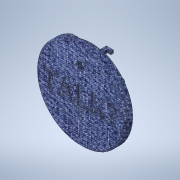
# Autodesk Inventor part: ButtonCap
Saved by Autodesk Inventor 2020.1 (Build 241239000, 239)
## iProperties
Created: 2019-10-05
Part Number: ButtonCap
Material: Plastic, Opaque Black
Document SubType Name: Modeling
Designer: Josiah
Density: 0.952 g/cm^3
Appearance: Denim - Blue
Author: Josiah
Autodesk Inventor part; units mm, degrees
ref_plane "YZ Plane" through (0, 0, 0) normal (1, 0, 0) x (0, 1, 0)
ref_plane "XZ Plane" through (0, 0, 0) normal (0, 1, 0) x (-1, 0, 0)
ref_plane "XY Plane" through (0, 0, 0) normal (0, 0, 1) x (1, 0, 0)
sketch "Sketch2" plane through (0, 0, 0) normal (0, 0, 1) x (1, 0, 0)
  arc A0 (-10.102, 26.1034) -> (10.102, 26.1034) centre (0, 0) ccw construction
  circle A1 centre (0, 0) radius 24.99 construction
  circle A2 centre (0, 0) radius 27.99
  constraints: 2 coincident, 1 centre point, 1 concentric, 3 other
extrude "BUTTON TOP" add sketch "Sketch2" along normal blind 3
chamfer "BUTTON TOP CHAMFER" distance 1 angle 45 1 edges at (-27.99, 0, 3)
sketch "Sketch3" plane through (0, 0, 0) normal (0, 0, -1) x (-1, 0, 0)
  circle A0 centre (0, 0) radius 24.99 projected
  line L0 (-10.102, 26.1034) -> (10.102, 26.1034) projected
  arc A1 (-10.102, 26.1034) -> (10.102, 26.1034) centre (0, 0) ccw projected
  point P0 (0, 0)
extrude "WALLS" add sketch "Sketch3" along normal blind 1.9
sketch "Sketch4" plane through (0, 0, 0) normal (0, 0, -1) x (-1, 0, 0)
  circle A0 centre (0, 0) radius 24.99 projected
  circle A1 centre (0, 0) radius 21.99
  point P0 (0, 0)
  dimension "d9" = 3
  constraints: 1 centre point
  measures "d9" radial gap between concentric circles of A0 A1
extrude "INNTER SHEATH" add sketch "Sketch4" along normal blind 4
sketch "Sketch5" plane through (0, 0, 0) normal (0, 0, -1) x (-1, 0, 0)
  circle A0 centre (0, 0) radius 3.5 construction
  circle A1 centre (0, 0) radius 4
  point P0 (0, 0)
  dimension "d12" = 0.5
  constraints: 1 centre point
  measures "d12" radial gap between concentric circles of A0 A1
extrude "BUTTON INDENT" cut sketch "Sketch5" against normal blind 1
sketch "Sketch6" plane through (0, 0, 0) normal (0, 0, -1) x (-1, 0, 0)
  circle A0 centre (-15, 10) radius 2.5 construction
  circle A1 centre (15, 10) radius 2.5 construction
  circle A2 centre (15, -10) radius 2.5 construction
  circle A3 centre (-15, -10) radius 2.5 construction
  circle A4 centre (-15, 10) radius 2.4
  circle A5 centre (15, 10) radius 2.4
  circle A6 centre (15, -10) radius 2.4
  circle A7 centre (-15, -10) radius 2.4
  point P0 (0, 0)
  dimension "d15" = 0.1
  dimension "d16" = 0.1
  dimension "d17" = 0.1
  dimension "d18" = 0.1
  constraints: 4 centre point
  measures "d15" radial gap between concentric circles of A1 A5
  measures "d16" radial gap between concentric circles of A2 A6
  measures "d17" radial gap between concentric circles of A3 A7
  measures "d18" radial gap between concentric circles of A0 A4
extrude "BUTTON-PINS" add sketch "Sketch6" along normal blind 8
fillet "PIN-FILLET" radius 0.5 4 edges at (17.4, 10, -8) (-12.6, 10, -8) (17.4, -10, -8) (-12.6, -10, -8)
sketch "Sketch7" plane through (0, 0, 0) normal (0, 0, -1) x (-1, 0, 0)
  line L0 (-9, 21.1034) -> (-8.5703, 21.1034) construction
  line L1 (-8.5703, 21.1034) -> (-6.6338, 21.1034) construction
  line L2 (-6.6338, 21.1034) -> (-5.6655, 21.1034) construction
  line L3 (-5.6655, 21.1034) -> (-4.602, 21.1034) construction
  circle A0 centre (0, 0) radius 24.99 construction
  line L4 (-9, 23.3131) -> (-9, 21.1034) construction
  line L5 (-8.702, 21.2034) -> (-4.302, 21.2034)
  line L6 (-4.302, 21.2034) -> (-4.302, 23.2034)
  line L7 (-4.302, 23.2034) -> (-8.702, 23.2034)
  line L8 (-8.702, 23.2034) -> (-8.702, 21.2034)
  point P0 (0, 0)
  dimension "d22" = 2
  dimension "d23" = 4.4
  dimension "d24" = 0.1
  dimension "d25" = 0.3
  constraints: 8 end point, 2 parallel, 1 horizontal, 1 perpendicular, 1 other
  measures "d22" distance of L5.end L6.end
  measures "d23" distance of L6.end L7.end
  measures "d24" distance between parallel lines of L5 L3
  measures "d25" distance from line of L6 L3.end
extrude "LOCK BLOCK" add sketch "Sketch7" along normal blind 9
sketch "Sketch8" plane through (4.302, 23.2034, -4) normal (0, 1, 0) x (1, 0, 0)
  line L0 (4.4, 0) -> (0, 0) projected
  line L1 (4.4, 0) -> (4.4, 5) projected
  line L2 (0, 5) -> (4.4, 5) projected
  line L3 (0, 0) -> (0, 5) projected
  line L4 (4.4, 3.5) -> (2.2, 3.5)
  line L5 (2.2, 3.5) -> (2.2, 0)
  line L6 (2.2, 0) -> (4.4, 0)
  line L7 (4.4, 0) -> (4.4, 3.5)
  circle A0 centre (3.3, 2.4) radius 1 construction
  circle A1 centre (3.3, 2.4) radius 0.9
  point P0 (-4.302, -4)
  dimension "d28" = 0.1
  dimension "d29" = 0.2
  dimension "d32" = 0.2
  dimension "d33" = 1.5
  dimension "d44" = 0
  constraints: 8 end point, 2 parallel, 1 centre point, 1 horizontal, 1 perpendicular
  measures "d28" radial gap between concentric circles of A0 A1
  measures "d29" distance edge to line of A1 L5
  measures "d32" distance edge to line of A1 L4
  measures "d33" distance edge to line of A1 L6
  measures "d44" distance between parallel lines of L1 L7
extrude "LOCK HOLE" cut sketch "Sketch8" against normal up to next contours L0 L5 L4 L1 | A1
fillet "LOCK HOLE FILLET" radius 0.2 2 edges at (6.502, 22.2034, -7.5) (6.502, 22.2034, -4)
sketch "Sketch9" plane through (0, 0, 3) normal (0, 0, 1) x (1, 0, 0)
  circle A0 centre (0, 16) radius 2.5
  point P0 (0, 0)
  point P1 (0, 0)
  dimension "d37" = 5
  dimension "d38" = 0
  dimension "d39" = 16
  constraints: 1 centre point, 1 coincident, 2 other
  measures "d37" diameter of A0
  measures "d38" horizontal distance of point (0, 0) A0.centre
  measures "d39" distance of A0.centre point (0, 0)
extrude "LED HOLE" cut sketch "Sketch9" against normal up to next
sketch "Sketch10" plane through (0, 0, 3) normal (0, 0, 1) x (1, 0, 0)
  circle A0 centre (0, 16) radius 2.5 projected
  circle A1 centre (0, 0) radius 26.99 projected
  line L0 (-23.4481, 5.4662) -> (19.1517, 5.4662) construction
  line L1 (19.1517, 5.4662) -> (19.1517, -6.0554) construction
  line L2 (19.1517, -6.0554) -> (-23.4481, -6.0554) construction
  line L3 (-23.4481, -6.0554) -> (-23.4481, 5.4662) construction
  line L4 (-20.1058, -6.0627) -> (-20.1058, 3.0854)
  line L5 (-20.1058, 3.0854) -> (-23.4481, 3.0854)
  line L6 (-23.4481, 3.0854) -> (-23.4481, 5.2373)
  line L7 (-23.4481, 5.2373) -> (-13.9246, 5.2373)
  line L8 (-13.9246, 5.2373) -> (-13.9246, 3.0854)
  line L9 (-13.9246, 3.0854) -> (-17.267, 3.0854)
  line L10 (-17.267, 3.0854) -> (-17.267, -6.0627)
  line L11 (-17.267, -6.0627) -> (-20.1058, -6.0627)
  line L12 (-13.9796, -6.0627) -> (-10.161, 5.2373)
  line L13 (-10.161, 5.2373) -> (-7.0659, 5.2373)
  line L14 (-7.0659, 5.2373) -> (-3.2473, -6.0627)
  line L15 (-3.2473, -6.0627) -> (-6.1685, -6.0627)
  line L16 (-6.1685, -6.0627) -> (-6.8736, -3.7551)
  line L17 (-6.8736, -3.7551) -> (-10.4266, -3.7551)
  line L18 (-10.4266, -3.7551) -> (-11.1408, -6.0627)
  line L19 (-11.1408, -6.0627) -> (-13.9796, -6.0627)
  line L20 (-7.4963, -1.7039) -> (-8.6501, 2.0323)
  line L21 (-8.6501, 2.0323) -> (-9.813, -1.7039)
  line L22 (-9.813, -1.7039) -> (-7.4963, -1.7039)
  line L23 (5.4154, -6.0627) -> (-2.121, -6.0627)
  line L24 (-2.121, -6.0627) -> (-2.121, 5.2373)
  line L25 (-2.121, 5.2373) -> (0.7177, 5.2373)
  line L26 (0.7177, 5.2373) -> (0.7177, -3.9107)
  line L27 (0.7177, -3.9107) -> (5.4154, -3.9107)
  line L28 (5.4154, -3.9107) -> (5.4154, -6.0627)
  line L29 (16.6696, -6.0627) -> (13.2357, -6.0627)
  line L30 (13.2357, -6.0627) -> (10.168, -1.4749)
  line L31 (10.168, -1.4749) -> (9.6094, -2.2441)
  line L32 (9.6094, -2.2441) -> (9.6094, -6.0627)
  line L33 (9.6094, -6.0627) -> (6.7707, -6.0627)
  line L34 (6.7707, -6.0627) -> (6.7707, 5.2373)
  line L35 (6.7707, 5.2373) -> (9.6094, 5.2373)
  line L36 (9.6094, 5.2373) -> (9.6094, 0.1917)
  line L37 (9.6094, 0.1917) -> (13.2357, 5.2373)
  line L38 (13.2357, 5.2373) -> (16.5048, 5.2373)
  line L39 (16.5048, 5.2373) -> (12.4756, -0.0098)
  line L40 (12.4756, -0.0098) -> (16.6696, -6.0627)
  spline S0 degree 2 poles (24.6455, 2.481) (24.6455, 1.7301) (24.1968, 0.5397) (23.7848, 0.1001) knots 0 0 0 1 2 2 2
  spline S1 degree 2 poles (23.7848, 0.1001) (23.391, -0.3303) (22.2555, -1.0079) (21.5596, -1.2918) knots 0 0 0 1 2 2 2
  line L41 (21.5596, -1.2918) -> (21.5596, -3.0225)
  line L42 (21.5596, -3.0225) -> (18.9681, -3.0225)
  line L43 (18.9681, -3.0225) -> (18.9681, -0.4768)
  spline S2 degree 2 poles (18.9681, -0.4768) (19.3893, -0.3669) (20.4332, 0.0269) (20.827, 0.3107) knots 0 0 0 1 2 2 2
  spline S3 degree 2 poles (20.827, 0.3107) (21.2391, 0.6129) (21.7702, 1.4004) (21.7702, 1.9407) knots 0 0 0 1 2 2 2
  spline S4 degree 2 poles (21.7702, 1.9407) (21.7702, 2.6916) (20.8178, 3.3692) (19.9662, 3.3692) knots 0 0 0 1 2 2 2
  spline S5 degree 2 poles (19.9662, 3.3692) (19.3252, 3.3692) (17.8967, 2.8106) (17.4846, 2.5268) knots 0 0 0 1 2 2 2
  line L44 (17.4846, 2.5268) -> (17.2648, 2.5268)
  line L45 (17.2648, 2.5268) -> (17.2648, 4.8161)
  spline S6 degree 2 poles (17.2648, 4.8161) (17.7502, 5.0267) (19.6182, 5.4662) (20.6896, 5.4662) knots 0 0 0 1 2 2 2
  spline S7 degree 2 poles (20.6896, 5.4662) (21.642, 5.4662) (23.1071, 5.0175) (23.6199, 4.6146) knots 0 0 0 1 2 2 2
  spline S8 degree 2 poles (23.6199, 4.6146) (24.1236, 4.2117) (24.6455, 3.1311) (24.6455, 2.481) knots 0 0 0 1 2 2 2
  line L46 (21.7702, -6.0627) -> (18.7849, -6.0627)
  line L47 (18.7849, -6.0627) -> (18.7849, -4.0573)
  line L48 (18.7849, -4.0573) -> (21.7702, -4.0573)
  line L49 (21.7702, -4.0573) -> (21.7702, -6.0627)
  point P0 (0, 0)
  constraints: 2 other
emboss "TALK? TEXT" sketch "Sketch10" operation cut depth 1 direction (0, 0, -1) contours L4 L5 L6 L7 L8 L9 L10 L11 | L12 L13 L14 L15 L16 L17 L18 L19 | L23 L24 L25 L26 L27 L28 | L29 L30 L31 L32 L33 L34 L35 L36 L37 L38 L39 L40 | S0 S1 L41 L42 L43 S2 S3 S4 S5 L44 L45 S6 S7 S8 | L46 L47 L48 L49
body "Solid2"
